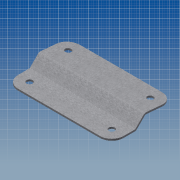
# Autodesk Inventor part: J009836
Saved by Autodesk Inventor 2020.3 (Build 243373000, 373)
## iProperties
RuleStatus: InUse
AfterDocSave0: file://Part Number Cleaner
Created: 2021-03-27
Material: STAINLESS STEEL, 316
Catalog Web Link: https://www.janelia.org/
Vendor: HHMI: JRC - ID&F
Document SubType Name: Sheet Metal
Designer: talbotj
Density: 8 g/cm^3
Sheet Metal Rule: Default
Appearance: Metal-Steel (Stainless, Brushed)
Flat Pattern Width: 3.54919 cm
Flat Pattern Length: 5.715 cm
Flat Pattern Area: 20.2836 cm^2
Sheet Metal Width: 1.397 in
Sheet Metal Length: 2.250 in
Sheet Metal Area: 3.144 in^2
Part Number: J009836
Description: N/A
Project: N/A
DESIGN DEPARTMENT: HHMI: JRC - ID&F
SPECIAL FINISH: N/A
LAB/DEPT: VIVARIUM (SHARED RESOURCES)
REQUESTING SCIENTIST: COX, JAMES
SURFACE ROUGHNESS: N/A
Thickness: 0.036 in
ALTERED ITEM PART NUMBER: N/A
ALTERED ITEM VENDOR: N/A
ALTERED ITEM DESCRIPTION: N/A
PART NUMBER - LEGACY: N/A
Author: talbotj
Revision Number: -
Autodesk Inventor part; units mm, degrees
ref_plane "YZ Plane" through (0, 0, 0) normal (1, 0, 0) x (0, 1, 0)
ref_plane "XZ Plane" through (0, 0, 0) normal (0, 1, 0) x (-1, 0, 0)
ref_plane "XY Plane" through (0, 0, 0) normal (0, 0, 1) x (1, 0, 0)
sketch "Sketch4" plane through (0, 0, 0) normal (0, 1, 0) x (1, 0, 0)
  line L0 (22.225, -12.319) -> (-22.225, -12.319) construction
  line L1 (0, 12.7356) -> (0, -16.4948) construction
  point P0 (0, 0)
  point P1 (22.225, 8.5598)
  point P2 (-22.225, 8.5598)
  dimension "d23" = 44.45
  dimension "d25" = 20.8788
  dimension "d26" = 12.319
  constraints: 2 end point, 2 vertical alignment, 1 horizontal, 1 horizontal alignment, 1 symmetric about line
  measures "d23" distance of L0.start L0.end
  measures "d25" distance from line of point (22.225, 8.56) L0
  measures "d26" distance from line of point (0, 0) L0
sketch "Sketch1" plane through (0, 0, 0) normal (0, 1, 0) x (-1, 0, 0)
  line L0 (28.575, 18.669) -> (-28.575, 18.669)
  line L1 (-28.575, 18.669) -> (-28.575, 5.969)
  line L2 (-28.575, 5.969) -> (28.575, 5.969)
  line L3 (28.575, 5.969) -> (28.575, 18.669)
  line L4 (28.575, 18.669) -> (-28.575, 5.969) construction
  line L5 (-28.575, 18.669) -> (28.575, 5.969) construction
  line L6 (0, 3.429) -> (0, 21.209)
  point P0 (0, 12.319)
  point P1 (-22.225, 12.319)
  point P2 (0, 12.319)
  point P3 (0, 12.319)
  dimension "d27" = 6.35
  dimension "d28" = 6.35
  dimension "d29" = 6.35
  measures "d27" distance from line of L0 point (-22.225, 12.319)
  measures "d28" distance from line of L1 point (-22.225, 12.319)
  measures "d29" distance from line of L2 point (-22.225, 12.319)
extrude "Plate1" add sketch "Sketch1" along normal blind 0.9144
sketch "Sketch2" plane through (-28.575, 0.9144, 5.969) normal (0, -0.7071068, -0.7071068) x (1, 0, 0)
  line L0 (57.15, 0) -> (0, 0)
  line L1 (0, 0) -> (0, -6.8054)
  line L2 (0, -6.8054) -> (57.15, -6.8054)
  line L3 (57.15, -6.8054) -> (57.15, 0)
  constraints: 6 end point, 1 horizontal, 1 perpendicular, 1 vertical
edge flange "Flange1" height 5.08 angle 45 thickness 0.9144 bend radius 0.762 thickness toward (0, -0.7071068, -0.7071068) relief tear relief width 0.9144 relief depth 0.4572 edges at (0, 0.9144, 5.969) wall of the first edge with corners at (28.575, 0.9144, 5.969) (-28.575, 0.9144, 5.969) (-28.575, 5.7266, 1.1568) (28.575, 5.7266, 1.1568)
bend "Bend1"
corner "Corner1"
sketch "Sketch3" plane through (28.575, 5.08, 0.5102) normal (0, 0.9961947, -0.0871557) x (-1, 0, 0)
  line L0 (57.15, 0) -> (0, 0)
  line L1 (0, 0) -> (0, -15.3978)
  line L2 (0, -15.3978) -> (57.15, -15.3978)
  line L3 (57.15, -15.3978) -> (57.15, 0)
  constraints: 6 end point, 1 horizontal, 1 perpendicular, 1 vertical
edge flange "Flange2" height 15.8242 angle 50 thickness 0.9144 bend radius 0.762 thickness toward (0, 0.9961947, -0.0871557) relief tear relief width 0.9144 relief depth 0.4572 edges at (0, 5.08, 0.5102) wall of the first edge with corners at (-28.575, 5.08, 0.5102) (28.575, 5.08, 0.5102) (28.575, 3.738, -14.829) (-28.575, 3.738, -14.829)
bend "Bend2"
corner "Corner2"
hole "Hole1" at (22.225, 0, 12.319) at (-22.225, 0, 12.319) at (22.225, 0, -8.5598) at (-22.225, 0, -8.5598) direction (0, 1, 0) diameter 3.2512 end through all
fillet "Corner Round1" radius 6.35 4 edges at (28.575, 4.1935, -14.8688) (-28.575, 4.1935, -14.8688) (-28.575, 0.4572, 18.669) (28.575, 0.4572, 18.669)
equation "\"d28\" = d27"
equation "\"d35\" = Thickness"
equation "\"d2\" = Thickness"
equation "\"d3\" = BendReliefWidth"
equation "\"d4\" = BendReliefDepth"
equation "\"d5\" = MinimumRemnant"
equation "\"d6\" = TransitionRadius"
equation "\"d9\" = BendRadius"
equation "\"d10\" = CornerReliefSize"
equation "\"d11\" = GapSize"
equation "\"d12\" = JacobiRadiusSize"
equation "\"d13\" = BendReliefWidth"
equation "\"d14\" = BendReliefDepth"
equation "\"d15\" = MinimumRemnant"
equation "\"d16\" = TransitionRadius"
equation "\"d19\" = BendRadius"
equation "\"d20\" = CornerReliefSize"
equation "\"d21\" = GapSize"
equation "\"d22\" = JacobiRadiusSize"
equation "\"BendReliefWidth\" = Thickness"
equation "\"BendReliefDepth\" = 0.5 * Thickness"
equation "\"CornerReliefSize\" = 4 * Thickness"
equation "\"MinimumRemnant\" = 2 * Thickness"
equation "\"TransitionRadius\" = BendRadius"
equation "\"JacobiRadiusSize\" = BendRadius"
equation "\"GapSize\" = Thickness"
equation "\"Thickness\" = 0.9144"
equation "\"BendRadius\" = 0.762"
body "Solid1"
